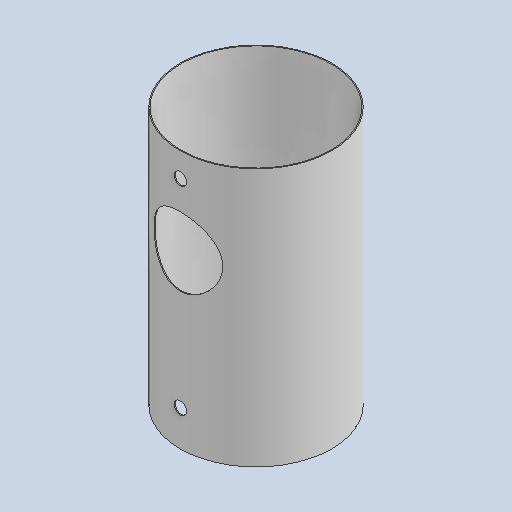
# Autodesk Inventor part: TZS 0902 SHELL
Saved by Autodesk Inventor 2025 (Build 290162010, 162A)
## iProperties
Created: 2025-02-11
Part Number: TZS 0902 SHELL
Material: Steel
Document SubType Name: Sheet Metal
Designer: pokla
Mass: 309189 g
Surface Area: 132135 cm^2
Volume: 39387.1 cm^3
Density: 7.85 g/cm^3
Sheet Metal Rule: Default_mm
Sheet Metal Width: 0,000 mm
Sheet Metal Length: 0,000 mm
Sheet Metal Area: 0,000 mm^2
Appearance: Default
Author: pokla
Autodesk Inventor part; units mm, degrees
sketch "floor angle sketch" plane through (0, 0, 0) normal (0, 0, 1) x (1, 0, 0)
  line L0 (0, 0) -> (0, -240.1382) construction
  line L1 (0, 0) -> (0, -870)
  line L2 (-332.3402, -332.3402) -> (332.3402, 332.3402) construction
  circle A0 centre (0, 0) radius 470 construction
  line L3 (0, 0) -> (0, -670)
  line L4 (-38, -670) -> (38, -670)
  line L5 (-213, -870) -> (213, -870)
  line L6 (0, 0) -> (-263.3555, -723.5633)
  line L7 (0, 0) -> (0, -570)
  line L8 (-38, -570) -> (38, -570)
  line L9 (-324.4355, -701.332) -> (-202.2755, -745.7946)
  dimension "d51" = 940
  dimension "d52" = 45
  dimension "d54" = 0
  dimension "d55" = 0
  dimension "d56" = 426
  dimension "d58" = 76
  dimension "d59" = 76
  dimension "d60" = 0
  dimension "d61" = 570
  dimension "d62" = 130
  dimension "d63" = 20
  dimension "d64" = 670
  dimension "d65" = 770
  dimension "d66" = 870
  constraints: 20 end point, 5 midpoint, 4 perpendicular, 1 coincident, 1 vertical, 3 other
  measures "d51" distance of L2.start L2.end
  measures "d52" angle of L0 L2
  measures "d54" distance between parallel lines of L0 L1
  measures "d55" distance between parallel lines of L0 L3
  measures "d56" distance of L5.start L5.end
  measures "d58" distance of L4.start L4.end
  measures "d59" distance of L8.start L8.end
  measures "d60" distance between parallel lines of L0 L7
  measures "d61" distance of L3.start L7.end
  measures "d62" distance of L9.start L9.end
  measures "d63" angle of L0 L6
  measures "d64" distance of L3.start L3.end
  measures "d65" distance of L3.start L6.end
  measures "d66" distance of L0.start L1.end
ref_plane "SHELL Plane" through (-332.3402, -332.3402, 0) normal (0.7071, -0.7071, 0) x (0.7071, 0.7071, 0)
ref_plane "ACCESS Plane" through (-213, -870, 0) normal (0, -1, 0) x (1, 0, 0)
ref_plane "OUTER Plane" through (-38, -670, 0) normal (0, -1, 0) x (1, 0, 0)
ref_plane "INNER Plane" through (-38, -570, 0) normal (0, -1, 0) x (1, 0, 0)
ref_plane "CHARGE Plane" through (-324.4355, -701.332, 0) normal (-0.342, -0.9397, 0) x (0.9397, -0.342, 0)
sketch "Sketch13" plane through (-332.3402, -332.3402, 0) normal (0.7071, -0.7071, 0) x (0.7071, 0.7071, 0)
  line L0 (470, 0) -> (470, 892.6829)
  line L1 (0, 0) -> (6, 0)
  line L2 (6, 0) -> (6, 1600)
  line L3 (6, 1600) -> (0, 1600)
  line L4 (0, 1600) -> (0, 0)
  dimension "d75" = 1600
  dimension "d76" = 6
  dimension "d77" = 940
  constraints: 10 end point, 2 parallel, 1 horizontal, 1 perpendicular, 1 vertical
  measures "d75" distance of L3.end L1.start
  measures "d76" distance between parallel lines of L2 L4
  measures "d77" diameter of L4 L0
revolve "Revolution2" add sketch "Sketch13" angle 359.9 about axis through (0, 0, 0) along (0, 0, 1)
sketch "Sketch14" plane through (-213, -870, 0) normal (0, -1, 0) x (1, 0, 0)
  circle A0 centre (213, 1060) radius 213
  line L0 (683, 1600) -> (-257, 1600) projected
  point P0 (213, 0)
  point P1 (-119.3402, 1600)
  point P2 (-119.9197, 1600)
  dimension "d80" = 426
  dimension "d93" = 540
  constraints: 1 centre point, 1 vertical alignment
  measures "d80" diameter of A0
  measures "d93" distance from line of L0 A0.centre
extrude "ACCESS" cut sketch "Sketch14" against normal up to next
sketch "Sketch15" plane through (-38, -570, 0) normal (0, -1, 0) x (1, 0, 0)
  circle A0 centre (38, 220) radius 38
  point P0 (38, 0)
  dimension "d84" = 76
  dimension "d85" = 220
  constraints: 1 centre point, 1 vertical alignment
  measures "d84" diameter of A0
  measures "d85" distance of A0.centre point (38, 0)
extrude "INNER" cut sketch "Sketch15" against normal up to next
sketch "Sketch16" plane through (-38, -670, 0) normal (0, -1, 0) x (1, 0, 0)
  circle A0 centre (38, 1450) radius 38
  line L0 (508, 1600) -> (-432, 1600) projected
  point P0 (38, 0)
  point P1 (-294.3402, 1600)
  point P2 (-294.9197, 1600)
  dimension "d89" = 76
  dimension "d92" = 150
  constraints: 1 centre point, 1 vertical alignment
  measures "d89" diameter of A0
  measures "d92" distance from line of L0 A0.centre
extrude "Extrusion9" cut sketch "Sketch16" against normal up to next
equation "\"BendRadius\" = Thickness"
equation "\"BendReliefWidth\" = Thickness"
equation "\"BendReliefDepth\" = 0.5 * Thickness"
equation "\"CornerReliefSize\" = 4 * Thickness"
equation "\"MinimumRemnant\" = 2 * Thickness"
equation "\"TransitionRadius\" = BendRadius"
equation "\"JacobiRadiusSize\" = BendRadius"
equation "\"GapSize\" = Thickness"
equation "\"Thickness\" = 6"
body "Solid2"
